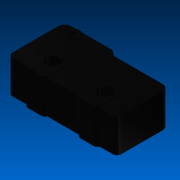
# Autodesk Inventor part: Omron SS-01GL2-E Microswitch Housing
Saved by Autodesk Inventor 2013 (Build 170138000, 138)
## iProperties
Created: 2012-05-23
Material: ABS Plastic
Document SubType Name: Modeling
Designer: sdarley
Density: 1 g/cm^3
Project: Microswitch - Omron SS-01GL2-E
Description: Omron SS-01GL2-E Microswitch Housing
Author: sdarley
Title: Omron SS-01GL2-E Microswitch Housing
Revision Number: 1
Autodesk Inventor part; units mm, degrees
ref_plane "YZ Plane" through (0, 0, 0) normal (1, 0, 0) x (0, 1, 0)
ref_plane "XZ Plane" through (0, 0, 0) normal (0, 1, 0) x (-1, 0, 0)
ref_plane "XY Plane" through (0, 0, 0) normal (0, 0, 1) x (1, 0, 0)
sketch "Sketch1" plane through (0, 0, 0) normal (0, 0, 1) x (1, 0, 0)
  line L0 (-9.75, 5.15) -> (-1, 5.15)
  line L1 (-1, 5.15) -> (0, 4.35)
  line L2 (0, 4.35) -> (10.1, 4.35)
  line L3 (10.1, 4.35) -> (10.1, -5.15)
  line L4 (10.1, -5.15) -> (6.75, -5.15)
  line L5 (6.75, -5.15) -> (6.3375, -5.45)
  line L6 (6.3375, -5.45) -> (3.5375, -5.45)
  line L7 (3.5375, -5.45) -> (3.125, -5.15)
  line L8 (3.125, -5.15) -> (-2.775, -5.15)
  line L9 (-2.775, -5.15) -> (-3.1875, -5.45)
  line L10 (-3.1875, -5.45) -> (-5.9875, -5.45)
  line L11 (-5.9875, -5.45) -> (-6.4, -5.15)
  line L12 (-6.4, -5.15) -> (-9.75, -5.15)
  line L13 (-9.75, -5.15) -> (-9.75, 5.15)
  point P0 (0, 0)
  point P1 (-9.75, 0)
  dimension "d0" = 19.85
  dimension "d2" = 10.6
  dimension "d3" = 9.5
  dimension "d4" = 0.3
  dimension "d5" = 5.9
  dimension "d6" = 3.35
  dimension "d7" = 3.35
  dimension "d8" = 10.1
  dimension "d9" = 8.75
  dimension "d10" = 2.8
  constraints: 28 end point, 9 parallel, 4 horizontal alignment, 2 equal length, 1 horizontal, 1 midpoint, 1 perpendicular, 1 vertical alignment
  measures "d0" distance between parallel lines of L3 L13
  measures "d2" distance between parallel lines of L6 L0
  measures "d3" distance between parallel lines of L4 L2
  measures "d4" distance between parallel lines of L6 L4
  measures "d5" distance of L7.end L8.end
  measures "d6" distance from line of L3 L4.end
  measures "d7" distance from line of L11.end L13
  measures "d8" distance of L1.end L2.end
  measures "d9" distance of L0.start L0.end
  measures "d10" distance of L9.end L10.end
extrude "Extrusion1" add sketch "Sketch1" along normal mid plane 6.1
sketch "Sketch2" plane through (0, 0, 3.05) normal (0, 0, 1) x (1, 0, 0)
  line L0 (-1, 5.15) -> (-9.75, 5.15) projected
  line L1 (-9.75, 5.15) -> (-9.75, -5.15) projected
  line L2 (-9.75, -5.15) -> (-6.4, -5.15) projected
  line L3 (-6.4, -5.15) -> (-5.9875, -5.45) projected
  line L4 (-5.9875, -5.45) -> (-3.1875, -5.45) projected
  line L5 (-3.1875, -5.45) -> (-2.775, -5.15) projected
  line L6 (3.125, -5.15) -> (3.5375, -5.45) projected
  line L7 (3.5375, -5.45) -> (6.3375, -5.45) projected
  line L8 (6.3375, -5.45) -> (6.75, -5.15) projected
  line L9 (10.1, 4.35) -> (0, 4.35) projected
  line L10 (-6.4, -5.15) -> (-6.4, -2.2125)
  line L11 (-2.775, -2.2125) -> (-2.775, -5.15)
  line L12 (3.125, -5.15) -> (3.125, -2.2125)
  line L13 (6.75, -2.2125) -> (6.75, -5.15)
  arc A0 (-2.775, -2.2125) -> (-6.4, -2.2125) centre (-4.5875, -2.2125) ccw
  arc A1 (6.75, -2.2125) -> (3.125, -2.2125) centre (4.9375, -2.2125) ccw
  circle A2 centre (-6.95, 4.05) radius 1.1
  point P0 (0, 0)
  dimension "d14" = 4.75
  dimension "d15" = 2.2
  dimension "d16" = 1.7
  constraints: 8 end point, 5 tangent, 4 point on circle, 3 centre point, 3 parallel, 1 horizontal alignment, 1 perpendicular
  measures "d15" diameter of A2
  measures "d16" distance edge to line of A2 L1
extrude "Extrusion2" add sketch "Sketch2" along normal blind 0.15
mirror "Mirror1" about plane through (0, 0, 0) normal (0, 0, 1) of "Extrusion2"
sketch "Sketch3" plane through (0, 0, 3.2) normal (0, 0, 1) x (1, 0, 0)
  arc A0 (-2.775, -2.2125) -> (-6.4, -2.2125) centre (-4.5875, -2.2125) ccw projected
  line L0 (3.125, -5.15) -> (3.5375, -5.45) projected
  line L1 (3.5375, -5.45) -> (6.3375, -5.45) projected
  line L2 (6.3375, -5.45) -> (6.75, -5.15) projected
  line L3 (6.75, -5.15) -> (6.75, -2.2125) projected
  arc A1 (6.75, -2.2125) -> (3.125, -2.2125) centre (4.9375, -2.2125) ccw projected
  line L4 (3.125, -2.2125) -> (3.125, -5.15) projected
  circle A2 centre (-4.5875, -2.2125) radius 1.175
  circle A3 centre (4.9375, -2.2125) radius 1.175
  circle A4 centre (-6.95, 4.05) radius 1.1 projected
  line L5 (-7.35, 4.35) -> (-6.8, 4.35)
  line L6 (-6.8, 4.35) -> (-6.8, 3.35)
  line L7 (-6.8, 3.35) -> (-7.35, 3.35)
  line L8 (-7.35, 3.35) -> (-7.35, 4.35)
  line L9 (-1, 5.15) -> (-6.95, 5.15) projected
  line L10 (10.1, -5.15) -> (10.1, 4.35) projected
  point P0 (0, 0)
  dimension "d19" = 2.35
  dimension "d21" = 2.35
  dimension "d24" = 0.55
  dimension "d25" = 1
  dimension "d35" = 0.8
  dimension "d36" = 16.9
  constraints: 8 end point, 2 centre point, 2 coincident, 2 parallel, 1 horizontal, 1 perpendicular, 1 vertical alignment
  measures "d19" diameter of A2
  measures "d21" diameter of A3
  measures "d24" distance of L6.end L7.end
  measures "d25" distance of L5.end L6.end
  measures "d35" distance between parallel lines of L9 L5
  measures "d36" distance between parallel lines of L10 L6
extrude "Extrusion3" cut sketch "Sketch3" against normal through all contours A2 | A3 | L5 L6 L7 L8
sketch "Sketch4" plane through (-9.75, 5.15, 3.05) normal (0, 1, 0) x (1, 0, 0)
  line L0 (0, 6.1) -> (0, 0) projected
  line L1 (2.5, 5.2) -> (2.8, 5.2)
  line L2 (2.8, 5.2) -> (2.8, 0.9)
  line L3 (2.8, 0.9) -> (2.5, 0.9)
  line L4 (2.5, 0.9) -> (2.5, 5.2)
  line L5 (5.85, 4.65) -> (7.85, 4.65)
  line L6 (7.85, 4.65) -> (7.85, 1.45)
  line L7 (7.85, 1.45) -> (5.85, 1.45)
  line L8 (5.85, 1.45) -> (5.85, 4.65)
  point P0 (9.75, 3.05)
  point P1 (0, 3.05)
  point P2 (2.5, 3.05)
  point P3 (2.8, 3.05)
  point P4 (5.85, 3.05)
  dimension "d26" = 4.3
  dimension "d28" = 0.3
  dimension "d29" = 2.5
  dimension "d30" = 3.05
  dimension "d31" = 2
  dimension "d32" = 3.2
  constraints: 16 end point, 4 midpoint, 4 parallel, 2 horizontal, 2 horizontal alignment, 2 perpendicular
  measures "d26" distance of L3.end L1.start
  measures "d28" distance of L1.start L1.end
  measures "d29" distance between parallel lines of L0 L4
  measures "d30" distance between parallel lines of L8 L2
  measures "d31" distance between parallel lines of L8 L6
  measures "d32" distance of L5.end L6.end
extrude "Extrusion4" cut sketch "Sketch4" against normal up to surface (1.8 mm away)
fillet "Fillet1" radius 1.2 2 edges at (-9.75, 5.15, 0) (10.1, 4.35, 0)
fillet "Fillet2" radius 0.75 2 edges at (-9.75, -5.15, 0) (10.1, -5.15, 0)
fillet "Fillet3" radius 0.3 10 edges at (0, 4.35, 0) (-1, 5.15, 0) (-2.775, -5.15, 0) (-3.1875, -5.45, 0) (-5.9875, -5.45, 0) (-6.4, -5.15, 0) (3.125, -5.15, 0) (3.5375, -5.45, 0) (6.3375, -5.45, 0) (6.75, -5.15, 0)
sketch "Sketch5" plane through (0, 0, 3.05) normal (0, 0, 1) x (1, 0, 0)
  line L0 (-9, -5.15) -> (-6.4976, -5.15) projected
  line L1 (-2.6774, -5.15) -> (3.0274, -5.15) projected
  line L2 (-8.5414, -3.4705) -> (-7.3088, -3.4705) construction
  line L3 (-7.3088, -3.4705) -> (-7.3088, -5.15) construction
  line L4 (-7.3088, -5.15) -> (-8.5414, -5.15) construction
  line L5 (-8.5414, -5.15) -> (-8.5414, -3.4705) construction
  line L6 (0.0618, -3.4705) -> (2.7283, -3.4705) construction
  line L7 (2.7283, -3.4705) -> (2.7283, -5.15) construction
  line L8 (2.7283, -5.15) -> (0.0618, -5.15) construction
  line L9 (0.0618, -5.15) -> (0.0618, -3.4705) construction
  line L10 (7.3318, -3.4705) -> (9.7732, -3.4705) construction
  line L11 (9.7732, -3.4705) -> (9.7732, -5.15) construction
  line L12 (9.7732, -5.15) -> (7.3318, -5.15) construction
  line L13 (7.3318, -5.15) -> (7.3318, -3.4705) construction
  spline S0 degree 2 poles (-7.8527, -4.9205) (-7.9889, -4.9205) (-8.2192, -4.8286) (-8.3032, -4.7367) knots 0 0 0 1 2 2 2
  spline S1 degree 2 poles (-8.3032, -4.7367) (-8.3871, -4.6459) (-8.479, -4.3736) (-8.479, -4.1966) knots 0 0 0 1 2 2 2
  spline S2 degree 2 poles (-8.479, -4.1966) (-8.479, -4.0208) (-8.3894, -3.7598) (-8.3043, -3.6634) knots 0 0 0 1 2 2 2
  spline S3 degree 2 poles (-8.3043, -3.6634) (-8.2203, -3.5692) (-7.9912, -3.4705) (-7.8493, -3.4705) knots 0 0 0 1 2 2 2
  spline S4 degree 2 poles (-7.8493, -3.4705) (-7.779, -3.4705) (-7.6553, -3.491) (-7.6032, -3.5068) knots 0 0 0 1 2 2 2
  spline S5 degree 2 poles (-7.6032, -3.5068) (-7.5578, -3.5216) (-7.4636, -3.5636) (-7.4171, -3.5885) knots 0 0 0 1 2 2 2
  line L14 (-7.4171, -3.5885) -> (-7.4171, -3.8132)
  line L15 (-7.4171, -3.8132) -> (-7.4318, -3.8132)
  spline S6 degree 2 poles (-7.4318, -3.8132) (-7.4568, -3.7905) (-7.5339, -3.7269) (-7.5895, -3.6963) knots 0 0 0 1 2 2 2
  spline S7 degree 2 poles (-7.5895, -3.6963) (-7.6429, -3.6668) (-7.7688, -3.6294) (-7.8505, -3.6294) knots 0 0 0 1 2 2 2
  spline S8 degree 2 poles (-7.8505, -3.6294) (-7.9401, -3.6294) (-8.1001, -3.7031) (-8.1602, -3.7735) knots 0 0 0 1 2 2 2
  spline S9 degree 2 poles (-8.1602, -3.7735) (-8.2192, -3.8449) (-8.285, -4.0616) (-8.285, -4.1966) knots 0 0 0 1 2 2 2
  spline S10 degree 2 poles (-8.285, -4.1966) (-8.285, -4.3407) (-8.2158, -4.5483) (-8.1557, -4.6198) knots 0 0 0 1 2 2 2
  spline S11 degree 2 poles (-8.1557, -4.6198) (-8.0967, -4.689) (-7.939, -4.7594) (-7.8505, -4.7594) knots 0 0 0 1 2 2 2
  spline S12 degree 2 poles (-7.8505, -4.7594) (-7.7699, -4.7594) (-7.6326, -4.7196) (-7.5793, -4.6901) knots 0 0 0 1 2 2 2
  spline S13 degree 2 poles (-7.5793, -4.6901) (-7.5283, -4.6606) (-7.4523, -4.5994) (-7.4307, -4.5778) knots 0 0 0 1 2 2 2
  line L16 (-7.4307, -4.5778) -> (-7.4171, -4.5778)
  line L17 (-7.4171, -4.5778) -> (-7.4171, -4.8002)
  spline S14 degree 2 poles (-7.4171, -4.8002) (-7.4636, -4.8217) (-7.5453, -4.8615) (-7.6032, -4.8796) knots 0 0 0 1 2 2 2
  spline S15 degree 2 poles (-7.6032, -4.8796) (-7.6644, -4.9) (-7.7688, -4.9205) (-7.8527, -4.9205) knots 0 0 0 1 2 2 2
  line L18 (1.2054, -4.9) -> (0.9966, -4.9)
  line L19 (0.9966, -4.9) -> (0.3772, -3.6929)
  line L20 (0.3772, -3.6929) -> (0.3772, -4.9)
  line L21 (0.3772, -4.9) -> (0.2036, -4.9)
  line L22 (0.2036, -4.9) -> (0.2036, -3.5)
  line L23 (0.2036, -3.5) -> (0.468, -3.5)
  line L24 (0.468, -3.5) -> (1.0318, -4.6085)
  line L25 (1.0318, -4.6085) -> (1.0318, -3.5)
  line L26 (1.0318, -3.5) -> (1.2054, -3.5)
  line L27 (1.2054, -3.5) -> (1.2054, -4.9)
  spline S16 degree 2 poles (2.4795, -3.66) (2.5589, -3.753) (2.6474, -4.0253) (2.6474, -4.2) knots 0 0 0 1 2 2 2
  spline S17 degree 2 poles (2.6474, -4.2) (2.6474, -4.3702) (2.5612, -4.6459) (2.4795, -4.7389) knots 0 0 0 1 2 2 2
  spline S18 degree 2 poles (2.4795, -4.7389) (2.3932, -4.8365) (2.1652, -4.9295) (2.0279, -4.9295) knots 0 0 0 1 2 2 2
  spline S19 degree 2 poles (2.0279, -4.9295) (1.8861, -4.9295) (1.6592, -4.8331) (1.5764, -4.7389) knots 0 0 0 1 2 2 2
  spline S20 degree 2 poles (1.5764, -4.7389) (1.4958, -4.6459) (1.4096, -4.3725) (1.4096, -4.2) knots 0 0 0 1 2 2 2
  spline S21 degree 2 poles (1.4096, -4.2) (1.4096, -4.0242) (1.497, -3.7564) (1.5775, -3.66) knots 0 0 0 1 2 2 2
  spline S22 degree 2 poles (1.5775, -3.66) (1.6592, -3.567) (1.8872, -3.4705) (2.0279, -3.4705) knots 0 0 0 1 2 2 2
  spline S23 degree 2 poles (2.0279, -3.4705) (2.1709, -3.4705) (2.4, -3.5704) (2.4795, -3.66) knots 0 0 0 1 2 2 2
  spline S24 degree 2 poles (2.4534, -4.2) (2.4534, -4.0616) (2.3932, -3.8472) (2.3388, -3.7769) knots 0 0 0 1 2 2 2
  spline S25 degree 2 poles (2.3388, -3.7769) (2.2832, -3.7042) (2.1266, -3.6316) (2.0291, -3.6316) knots 0 0 0 1 2 2 2
  spline S26 degree 2 poles (2.0291, -3.6316) (1.9281, -3.6316) (1.7761, -3.702) (1.7182, -3.7769) knots 0 0 0 1 2 2 2
  spline S27 degree 2 poles (1.7182, -3.7769) (1.6626, -3.8483) (1.6036, -4.0639) (1.6036, -4.2) knots 0 0 0 1 2 2 2
  spline S28 degree 2 poles (1.6036, -4.2) (1.6036, -4.4757) (1.8351, -4.7684) (2.0291, -4.7684) knots 0 0 0 1 2 2 2
  spline S29 degree 2 poles (2.0291, -4.7684) (2.2231, -4.7684) (2.4534, -4.4757) (2.4534, -4.2) knots 0 0 0 1 2 2 2
  line L28 (8.4754, -4.8955) -> (8.2666, -4.8955)
  line L29 (8.2666, -4.8955) -> (7.6472, -3.6884)
  line L30 (7.6472, -3.6884) -> (7.6472, -4.8955)
  line L31 (7.6472, -4.8955) -> (7.4736, -4.8955)
  line L32 (7.4736, -4.8955) -> (7.4736, -3.4955)
  line L33 (7.4736, -3.4955) -> (7.7379, -3.4955)
  line L34 (7.7379, -3.4955) -> (8.3018, -4.6039)
  line L35 (8.3018, -4.6039) -> (8.3018, -3.4955)
  line L36 (8.3018, -3.4955) -> (8.4754, -3.4955)
  line L37 (8.4754, -3.4955) -> (8.4754, -4.8955)
  spline S30 degree 2 poles (9.3058, -4.9205) (9.1697, -4.9205) (8.9394, -4.8286) (8.8554, -4.7367) knots 0 0 0 1 2 2 2
  spline S31 degree 2 poles (8.8554, -4.7367) (8.7715, -4.6459) (8.6796, -4.3736) (8.6796, -4.1966) knots 0 0 0 1 2 2 2
  spline S32 degree 2 poles (8.6796, -4.1966) (8.6796, -4.0208) (8.7692, -3.7598) (8.8543, -3.6634) knots 0 0 0 1 2 2 2
  spline S33 degree 2 poles (8.8543, -3.6634) (8.9382, -3.5692) (9.1674, -3.4705) (9.3092, -3.4705) knots 0 0 0 1 2 2 2
  spline S34 degree 2 poles (9.3092, -3.4705) (9.3796, -3.4705) (9.5032, -3.491) (9.5554, -3.5068) knots 0 0 0 1 2 2 2
  spline S35 degree 2 poles (9.5554, -3.5068) (9.6008, -3.5216) (9.695, -3.5636) (9.7415, -3.5885) knots 0 0 0 1 2 2 2
  line L38 (9.7415, -3.5885) -> (9.7415, -3.8132)
  line L39 (9.7415, -3.8132) -> (9.7267, -3.8132)
  spline S36 degree 2 poles (9.7267, -3.8132) (9.7018, -3.7905) (9.6246, -3.7269) (9.569, -3.6963) knots 0 0 0 1 2 2 2
  spline S37 degree 2 poles (9.569, -3.6963) (9.5157, -3.6668) (9.3898, -3.6294) (9.3081, -3.6294) knots 0 0 0 1 2 2 2
  spline S38 degree 2 poles (9.3081, -3.6294) (9.2185, -3.6294) (9.0585, -3.7031) (8.9984, -3.7735) knots 0 0 0 1 2 2 2
  spline S39 degree 2 poles (8.9984, -3.7735) (8.9394, -3.8449) (8.8736, -4.0616) (8.8736, -4.1966) knots 0 0 0 1 2 2 2
  spline S40 degree 2 poles (8.8736, -4.1966) (8.8736, -4.3407) (8.9428, -4.5483) (9.0029, -4.6198) knots 0 0 0 1 2 2 2
  spline S41 degree 2 poles (9.0029, -4.6198) (9.0619, -4.689) (9.2196, -4.7594) (9.3081, -4.7594) knots 0 0 0 1 2 2 2
  spline S42 degree 2 poles (9.3081, -4.7594) (9.3886, -4.7594) (9.5259, -4.7196) (9.5792, -4.6901) knots 0 0 0 1 2 2 2
  spline S43 degree 2 poles (9.5792, -4.6901) (9.6303, -4.6606) (9.7063, -4.5994) (9.7279, -4.5778) knots 0 0 0 1 2 2 2
  line L40 (9.7279, -4.5778) -> (9.7415, -4.5778)
  line L41 (9.7415, -4.5778) -> (9.7415, -4.8002)
  spline S44 degree 2 poles (9.7415, -4.8002) (9.695, -4.8217) (9.6133, -4.8615) (9.5554, -4.8796) knots 0 0 0 1 2 2 2
  spline S45 degree 2 poles (9.5554, -4.8796) (9.4942, -4.9) (9.3898, -4.9205) (9.3058, -4.9205) knots 0 0 0 1 2 2 2
  point P0 (0, 0)
  constraints: 3 horizontal alignment, 2 point on line, 6 other
extrude "Extrusion5" add sketch "Sketch5" along normal blind 0.05
sketch "Sketch6" plane through (0, 0, -3.05) normal (0, 0, -1) x (-1, 0, 0)
  arc A0 (-0.1052, 4.35) -> (0.0822, 4.4157) centre (-0.1052, 4.65) ccw projected
  line L0 (-0.0059, 4.3669) -> (7.1408, 4.3669) construction
  line L1 (7.1408, 4.3669) -> (7.1408, 2.1169) construction
  line L2 (7.1408, 2.1169) -> (-0.0059, 2.1169) construction
  line L3 (-0.0059, 2.1169) -> (-0.0059, 4.3669) construction
  line L4 (-10.1, 3.15) -> (-10.1, -4.4) projected
  line L5 (-9.35, -5.15) -> (-6.8476, -5.15) projected
  line L6 (-3.0274, -5.15) -> (2.6774, -5.15) projected
  line L7 (9.75, -4.4) -> (9.75, 3.95) projected
  line L8 (-9.1339, -3.4715) -> (-8.1314, -3.4715) construction
  line L9 (-8.1314, -3.4715) -> (-8.1314, -4.8125) construction
  line L10 (-8.1314, -4.8125) -> (-9.1339, -4.8125) construction
  line L11 (-9.1339, -4.8125) -> (-9.1339, -3.4715) construction
  line L12 (-2.1546, -3.4715) -> (-1.2541, -3.4715) construction
  line L13 (-1.2541, -3.4715) -> (-1.2541, -4.8125) construction
  line L14 (-1.2541, -4.8125) -> (-2.1546, -4.8125) construction
  line L15 (-2.1546, -4.8125) -> (-2.1546, -3.4715) construction
  line L16 (7.4519, -3.4715) -> (8.3839, -3.4715) construction
  line L17 (8.3839, -3.4715) -> (8.3839, -4.8125) construction
  line L18 (8.3839, -4.8125) -> (7.4519, -4.8125) construction
  line L19 (7.4519, -4.8125) -> (7.4519, -3.4715) construction
  line L20 (-8.9, -3.15) -> (-8.5, -3.15)
  line L21 (-8.5, -3.15) -> (-8.5, 0.2)
  line L22 (-8.5, 0.2) -> (-2, 0.2)
  line L23 (-8.9, -3.15) -> (-8.9, 0.6)
  line L24 (-8.9, 0.6) -> (-1.6, 0.6)
  line L25 (-0.0393, -1.1) -> (2.55, -1.1)
  line L26 (2.55, -1.1) -> (2.55, -1.5)
  line L27 (2.55, -1.5) -> (-0.1, -1.5)
  line L28 (5.8899, -5.45) -> (3.2851, -5.45) projected
  line L29 (-1.6, 0.6) -> (-1.6, -0.3)
  line L30 (-1.6, -0.3) -> (-1.5113, -0.3)
  line L31 (-1.5113, -0.3) -> (-1.8, -0.8)
  line L32 (-2, 0.2) -> (-2, -0.3)
  line L33 (-2, -0.3) -> (-2.0887, -0.3)
  line L34 (-2.0887, -0.3) -> (-1.8, -0.8)
  line L35 (-0.0393, -1.1) -> (-2.1313, -0.45)
  line L36 (-2.1313, -0.45) -> (-2.25, -0.832)
  line L37 (-2.25, -0.832) -> (-0.1, -1.5)
  line L38 (-3.6351, -5.45) -> (-6.2399, -5.45) projected
  line L39 (6.85, -1.1) -> (6.85, -1.5)
  line L40 (6.85, -1.5) -> (7.7, -1.5)
  line L41 (7.7, -1.5) -> (7.7, -3.15)
  line L42 (7.7, -3.15) -> (8.1, -3.15)
  line L43 (8.1, -3.15) -> (8.1, -1.1)
  line L44 (8.1, -1.1) -> (6.85, -1.1)
  line L45 (-1.6, -3.15) -> (-2, -3.15)
  line L46 (-2, -3.15) -> (-2, -2.333)
  line L47 (-2, -2.333) -> (-2.05, -2.333)
  line L48 (-2.05, -2.333) -> (-1.8, -1.9)
  line L49 (-1.8, -1.9) -> (-1.55, -2.333)
  line L50 (-1.55, -2.333) -> (-1.6, -2.333)
  line L51 (-1.6, -2.333) -> (-1.6, -3.15)
  line L52 (0.9178, 5.0843) -> (0.0822, 4.4157) projected
  circle A1 centre (-7.7959, 3.0628) radius 0.4188
  circle A2 centre (-7.7959, 3.0628) radius 0.7
  circle A3 centre (-3.3347, 3.0628) radius 0.4188
  circle A4 centre (-3.3347, 3.0628) radius 0.7
  line L53 (-6.98, 3.7628) -> (-6.98, 2.3628)
  line L54 (-6.98, 2.3628) -> (-6.7014, 2.3628)
  line L55 (-6.7014, 3.4816) -> (-6.7014, 2.3628)
  line L56 (-6.7014, 3.4816) -> (-6.3607, 3.4816)
  line L57 (-6.3607, 3.4816) -> (-6.3607, 2.3628)
  line L58 (-6.0774, 2.3628) -> (-6.0774, 3.4816)
  line L59 (-6.0774, 3.4816) -> (-5.8769, 3.4816)
  line L60 (-6.98, 3.7628) -> (-5.8746, 3.7628)
  line L61 (-6.3607, 2.3628) -> (-6.0774, 2.3628)
  line L62 (-5.7287, 2.3628) -> (-5.7287, 3.3334)
  line L63 (-5.7287, 2.3628) -> (-5.4364, 2.3628)
  line L64 (-5.4364, 2.3628) -> (-5.4364, 3.2892)
  line L65 (-5.272, 3.7628) -> (-5.272, 2.3628)
  line L66 (-5.272, 2.3628) -> (-4.9837, 2.3628)
  line L67 (-4.9837, 2.3628) -> (-4.9837, 3.5038)
  line L68 (-5.272, 3.7628) -> (-4.5256, 3.7628)
  line L69 (-4.4487, 2.8778) -> (-4.0366, 2.3628)
  line L70 (-4.3901, 2.3628) -> (-4.0366, 2.3628)
  line L71 (-4.3901, 2.3628) -> (-4.8491, 3.0137)
  line L72 (-4.9837, 3.5038) -> (-4.6228, 3.5038)
  arc A5 (-5.4364, 3.2892) -> (-5.8746, 3.7628) centre (-5.9114, 3.2892) ccw
  arc A6 (-5.7287, 3.3334) -> (-5.8769, 3.4816) centre (-5.8769, 3.3334) ccw
  arc A7 (-4.5825, 3.0628) -> (-4.6228, 3.5038) centre (-4.6228, 3.2815) ccw
  arc A8 (-4.4487, 2.8778) -> (-4.5256, 3.7628) centre (-4.5825, 3.312) ccw
  line L73 (-4.8491, 3.0137) -> (-4.5825, 3.0628)
  line L74 (-2.5151, 2.3628) -> (-2.5151, 2.443)
  line L75 (-2.5151, 2.443) -> (-2.5151, 3.7628)
  line L76 (-2.5151, 3.7628) -> (-1.836, 3.7628)
  line L77 (-2.5151, 2.3628) -> (-2.2307, 2.3628)
  line L78 (-2.2307, 3.5038) -> (-2.2307, 2.3628)
  line L79 (-2.2307, 3.5038) -> (-1.869, 3.5038)
  line L80 (-1.675, 2.3628) -> (-1.675, 3.3098)
  line L81 (-1.675, 2.3628) -> (-1.4257, 2.3628)
  line L82 (-1.4257, 2.3628) -> (-1.4257, 3.3525)
  arc A9 (-1.675, 3.3098) -> (-1.869, 3.5038) centre (-1.869, 3.3098) ccw
  arc A10 (-1.4257, 3.3525) -> (-1.836, 3.7628) centre (-1.836, 3.3525) ccw
  line L83 (0.0726, 3.3669) -> (0.0726, 4.3669)
  line L84 (0.0726, 4.3669) -> (0.2212, 4.3669)
  line L85 (0.2212, 4.3669) -> (0.3988, 3.6588)
  spline S0 degree 2 poles (0.3988, 3.6588) (0.4232, 3.5597) (0.4346, 3.511) knots 0 0 0 1 1 1
  spline S1 degree 2 poles (0.4346, 3.511) (0.4468, 3.5651) (0.4743, 3.671) knots 0 0 0 1 1 1
  line L86 (0.4743, 3.671) -> (0.6541, 4.3669)
  line L87 (0.6541, 4.3669) -> (0.7868, 4.3669)
  line L88 (0.7868, 4.3669) -> (0.7868, 3.3669)
  line L89 (0.7868, 3.3669) -> (0.6915, 3.3669)
  line L90 (0.6915, 3.3669) -> (0.6915, 4.2038)
  line L91 (0.6915, 4.2038) -> (0.4735, 3.3669)
  line L92 (0.4735, 3.3669) -> (0.3843, 3.3669)
  line L93 (0.3843, 3.3669) -> (0.1678, 4.2183)
  line L94 (0.1678, 4.2183) -> (0.1678, 3.3669)
  line L95 (0.1678, 3.3669) -> (0.0726, 3.3669)
  line L96 (0.8645, 3.3669) -> (1.1518, 4.3669)
  line L97 (1.1518, 4.3669) -> (1.2593, 4.3669)
  line L98 (1.2593, 4.3669) -> (1.5657, 3.3669)
  line L99 (1.5657, 3.3669) -> (1.4529, 3.3669)
  line L100 (1.4529, 3.3669) -> (1.366, 3.6695)
  line L101 (1.366, 3.6695) -> (1.052, 3.6695)
  line L102 (1.052, 3.6695) -> (0.9697, 3.3669)
  line L103 (0.9697, 3.3669) -> (0.8645, 3.3669)
  line L104 (1.0802, 3.777) -> (1.3355, 3.777)
  line L105 (1.3355, 3.777) -> (1.257, 4.0544)
  spline S2 degree 2 poles (1.257, 4.0544) (1.2212, 4.1809) (1.2037, 4.2617) knots 0 0 0 1 1 1
  spline S3 degree 2 poles (1.2037, 4.2617) (1.1884, 4.1657) (1.1633, 4.0712) knots 0 0 0 1 1 1
  line L106 (1.1633, 4.0712) -> (1.0802, 3.777)
  line L107 (1.645, 3.3669) -> (1.645, 4.3669)
  line L108 (1.645, 4.3669) -> (1.9034, 4.3669)
  spline S4 degree 2 poles (1.9034, 4.3669) (1.9903, 4.3669) (2.0368, 4.3524) knots 0 0 0 1 1 1
  spline S5 degree 2 poles (2.0368, 4.3524) (2.1008, 4.3326) (2.1465, 4.2808) knots 0 0 0 1 1 1
  spline S6 degree 2 poles (2.1465, 4.2808) (2.206, 4.2145) (2.2646, 4.0064) (2.2646, 3.8722) knots 0 0 0 1 2 2 2
  spline S7 degree 2 poles (2.2646, 3.8722) (2.2646, 3.7587) (2.225, 3.5826) (2.1625, 3.4675) (2.0886, 3.4012) (1.9834, 3.3669) (1.9156, 3.3669) knots 0 0 0 1 2 3 4 5 5 5
  line L109 (1.9156, 3.3669) -> (1.645, 3.3669)
  line L110 (1.7441, 3.4851) -> (1.9041, 3.4851)
  spline S8 degree 2 poles (1.9041, 3.4851) (1.9781, 3.4851) (2.0627, 3.5216) (2.0878, 3.5552) knots 0 0 0 1 2 2 2
  spline S9 degree 2 poles (2.0878, 3.5552) (2.1229, 3.6024) (2.1625, 3.761) (2.1625, 3.8745) knots 0 0 0 1 2 2 2
  spline S10 degree 2 poles (2.1625, 3.8745) (2.1625, 4.0315) (2.0855, 4.2) (2.0299, 4.2282) knots 0 0 0 1 2 2 2
  spline S11 degree 2 poles (2.0299, 4.2282) (1.9903, 4.2488) (1.9018, 4.2488) knots 0 0 0 1 1 1
  line L111 (1.9018, 4.2488) -> (1.7441, 4.2488)
  line L112 (1.7441, 4.2488) -> (1.7441, 3.4851)
  line L113 (2.4026, 3.3669) -> (2.4026, 4.3669)
  line L114 (2.4026, 4.3669) -> (2.9438, 4.3669)
  line L115 (2.9438, 4.3669) -> (2.9438, 4.2488)
  line L116 (2.9438, 4.2488) -> (2.5017, 4.2488)
  line L117 (2.5017, 4.2488) -> (2.5017, 3.9431)
  line L118 (2.5017, 3.9431) -> (2.9156, 3.9431)
  line L119 (2.9156, 3.9431) -> (2.9156, 3.825)
  line L120 (2.9156, 3.825) -> (2.5017, 3.825)
  line L121 (2.5017, 3.825) -> (2.5017, 3.4851)
  line L122 (2.5017, 3.4851) -> (2.9613, 3.4851)
  line L123 (2.9613, 3.4851) -> (2.9613, 3.3669)
  line L124 (2.9613, 3.3669) -> (2.4026, 3.3669)
  line L125 (3.4057, 3.3669) -> (3.4057, 4.3669)
  line L126 (3.4057, 4.3669) -> (3.5047, 4.3669)
  line L127 (3.5047, 4.3669) -> (3.5047, 3.3669)
  line L128 (3.5047, 3.3669) -> (3.4057, 3.3669)
  line L129 (3.6785, 3.3669) -> (3.6785, 4.3669)
  line L130 (3.6785, 4.3669) -> (3.7807, 4.3669)
  line L131 (3.7807, 4.3669) -> (4.1732, 3.5819)
  line L132 (4.1732, 3.5819) -> (4.1732, 4.3669)
  line L133 (4.1732, 4.3669) -> (4.2685, 4.3669)
  line L134 (4.2685, 4.3669) -> (4.2685, 3.3669)
  line L135 (4.2685, 3.3669) -> (4.1663, 3.3669)
  line L136 (4.1663, 3.3669) -> (3.7738, 4.152)
  line L137 (3.7738, 4.152) -> (3.7738, 3.3669)
  line L138 (3.7738, 3.3669) -> (3.6785, 3.3669)
  line L139 (0.0916, 2.1669) -> (0.0916, 3.1669)
  line L140 (0.0916, 3.1669) -> (0.1907, 3.1669)
  line L141 (0.1907, 3.1669) -> (0.1907, 2.1669)
  line L142 (0.1907, 2.1669) -> (0.0916, 2.1669)
  line L143 (0.3645, 2.1669) -> (0.3645, 3.1669)
  line L144 (0.3645, 3.1669) -> (0.4666, 3.1669)
  line L145 (0.4666, 3.1669) -> (0.8592, 2.3819)
  line L146 (0.8592, 2.3819) -> (0.8592, 3.1669)
  line L147 (0.8592, 3.1669) -> (0.9544, 3.1669)
  line L148 (0.9544, 3.1669) -> (0.9544, 2.1669)
  line L149 (0.9544, 2.1669) -> (0.8523, 2.1669)
  line L150 (0.8523, 2.1669) -> (0.4598, 2.952)
  line L151 (0.4598, 2.952) -> (0.4598, 2.1669)
  line L152 (0.4598, 2.1669) -> (0.3645, 2.1669)
  line L153 (1.1206, 2.1669) -> (1.1206, 3.1669)
  line L154 (1.1206, 3.1669) -> (1.379, 3.1669)
  spline S12 degree 2 poles (1.379, 3.1669) (1.4659, 3.1669) (1.5124, 3.1524) knots 0 0 0 1 1 1
  spline S13 degree 2 poles (1.5124, 3.1524) (1.5764, 3.1326) (1.6221, 3.0808) knots 0 0 0 1 1 1
  spline S14 degree 2 poles (1.6221, 3.0808) (1.6816, 3.0145) (1.7403, 2.8064) (1.7403, 2.6722) knots 0 0 0 1 2 2 2
  spline S15 degree 2 poles (1.7403, 2.6722) (1.7403, 2.5587) (1.7006, 2.3826) (1.6381, 2.2675) (1.5642, 2.2012) (1.459, 2.1669) (1.3912, 2.1669) knots 0 0 0 1 2 3 4 5 5 5
  line L155 (1.3912, 2.1669) -> (1.1206, 2.1669)
  line L156 (1.2197, 2.2851) -> (1.3797, 2.2851)
  spline S16 degree 2 poles (1.3797, 2.2851) (1.4537, 2.2851) (1.5383, 2.3216) (1.5634, 2.3552) knots 0 0 0 1 2 2 2
  spline S17 degree 2 poles (1.5634, 2.3552) (1.5985, 2.4024) (1.6381, 2.561) (1.6381, 2.6745) knots 0 0 0 1 2 2 2
  spline S18 degree 2 poles (1.6381, 2.6745) (1.6381, 2.8315) (1.5611, 3) (1.5055, 3.0282) knots 0 0 0 1 2 2 2
  spline S19 degree 2 poles (1.5055, 3.0282) (1.4659, 3.0488) (1.3775, 3.0488) knots 0 0 0 1 1 1
  line L157 (1.3775, 3.0488) -> (1.2197, 3.0488)
  line L158 (1.2197, 3.0488) -> (1.2197, 2.2851)
  spline S20 degree 2 poles (1.8454, 2.654) (1.8454, 2.9032) (2.0459, 3.1844) (2.2044, 3.1844) knots 0 0 0 1 2 2 2
  spline S21 degree 2 poles (2.2044, 3.1844) (2.3081, 3.1844) (2.4743, 3.0518) (2.5619, 2.8155) (2.5619, 2.6654) knots 0 0 0 1 2 3 3 3
  spline S22 degree 2 poles (2.5619, 2.6654) (2.5619, 2.5137) (2.4697, 2.2736) (2.3012, 2.1501) (2.2037, 2.1501) knots 0 0 0 1 2 3 3 3
  spline S23 degree 2 poles (2.2037, 2.1501) (2.0977, 2.1501) (1.9316, 2.2866) (1.8454, 2.5221) (1.8454, 2.654) knots 0 0 0 1 2 3 3 3
  spline S24 degree 2 poles (1.9476, 2.6524) (1.9476, 2.4718) (2.0932, 2.2637) (2.2029, 2.2637) knots 0 0 0 1 2 2 2
  spline S25 degree 2 poles (2.2029, 2.2637) (2.315, 2.2637) (2.4598, 2.4733) (2.4598, 2.6669) knots 0 0 0 1 2 2 2
  spline S26 degree 2 poles (2.4598, 2.6669) (2.4598, 2.7889) (2.398, 2.971) (2.2791, 3.0709) (2.2044, 3.0709) knots 0 0 0 1 2 3 3 3
  spline S27 degree 2 poles (2.2044, 3.0709) (2.0993, 3.0709) (1.9476, 2.878) (1.9476, 2.6524) knots 0 0 0 1 2 2 2
  line L159 (2.6892, 2.1669) -> (2.6892, 3.1669)
  line L160 (2.6892, 3.1669) -> (2.7913, 3.1669)
  line L161 (2.7913, 3.1669) -> (3.1839, 2.3819)
  line L162 (3.1839, 2.3819) -> (3.1839, 3.1669)
  line L163 (3.1839, 3.1669) -> (3.2791, 3.1669)
  line L164 (3.2791, 3.1669) -> (3.2791, 2.1669)
  line L165 (3.2791, 2.1669) -> (3.177, 2.1669)
  line L166 (3.177, 2.1669) -> (2.7845, 2.952)
  line L167 (2.7845, 2.952) -> (2.7845, 2.1669)
  line L168 (2.7845, 2.1669) -> (2.6892, 2.1669)
  line L169 (3.4476, 2.1669) -> (3.4476, 3.1669)
  line L170 (3.4476, 3.1669) -> (3.9887, 3.1669)
  line L171 (3.9887, 3.1669) -> (3.9887, 3.0488)
  line L172 (3.9887, 3.0488) -> (3.5467, 3.0488)
  line L173 (3.5467, 3.0488) -> (3.5467, 2.7431)
  line L174 (3.5467, 2.7431) -> (3.9605, 2.7431)
  line L175 (3.9605, 2.7431) -> (3.9605, 2.625)
  line L176 (3.9605, 2.625) -> (3.5467, 2.625)
  line L177 (3.5467, 2.625) -> (3.5467, 2.2851)
  line L178 (3.5467, 2.2851) -> (4.0063, 2.2851)
  line L179 (4.0063, 2.2851) -> (4.0063, 2.1669)
  line L180 (4.0063, 2.1669) -> (3.4476, 2.1669)
  line L181 (4.1107, 2.4886) -> (4.2044, 2.4992)
  spline S28 degree 2 poles (4.2044, 2.4992) (4.2113, 2.4238) (4.2593, 2.3277) (4.3614, 2.2683) (4.4255, 2.2683) knots 0 0 0 1 2 3 3 3
  spline S29 degree 2 poles (4.4255, 2.2683) (4.4819, 2.2683) (4.5688, 2.3133) (4.6107, 2.3918) (4.6107, 2.4383) knots 0 0 0 1 2 3 3 3
  spline S30 degree 2 poles (4.6107, 2.4383) (4.6107, 2.4855) (4.5688, 2.5556) (4.5223, 2.5793) knots 0 0 0 1 2 2 2
  spline S31 degree 2 poles (4.5223, 2.5793) (4.4918, 2.5953) (4.286, 2.6616) (4.2448, 2.6913) knots 0 0 0 1 2 2 2
  spline S32 degree 2 poles (4.2448, 2.6913) (4.1915, 2.7286) (4.1389, 2.8399) (4.1389, 2.9085) knots 0 0 0 1 2 2 2
  spline S33 degree 2 poles (4.1389, 2.9085) (4.1389, 2.9847) (4.2029, 3.1158) (4.3264, 3.1844) (4.4018, 3.1844) knots 0 0 0 1 2 3 3 3
  spline S34 degree 2 poles (4.4018, 3.1844) (4.4849, 3.1844) (4.6122, 3.1128) (4.6808, 2.9733) (4.6831, 2.8857) knots 0 0 0 1 2 3 3 3
  line L182 (4.6831, 2.8857) -> (4.5878, 2.8758)
  spline S35 degree 2 poles (4.5878, 2.8758) (4.5802, 2.971) (4.4918, 3.0678) (4.4057, 3.0678) knots 0 0 0 1 2 2 2
  spline S36 degree 2 poles (4.4057, 3.0678) (4.3165, 3.0678) (4.2342, 2.9794) (4.2342, 2.9177) knots 0 0 0 1 2 2 2
  spline S37 degree 2 poles (4.2342, 2.9177) (4.2342, 2.8636) (4.2631, 2.8285) knots 0 0 0 1 1 1
  spline S38 degree 2 poles (4.2631, 2.8285) (4.2921, 2.7942) (4.5329, 2.721) (4.5779, 2.6936) knots 0 0 0 1 2 2 2
  spline S39 degree 2 poles (4.5779, 2.6936) (4.6435, 2.6532) (4.706, 2.5297) (4.706, 2.4497) knots 0 0 0 1 2 2 2
  spline S40 degree 2 poles (4.706, 2.4497) (4.706, 2.3697) (4.6374, 2.2286) (4.5093, 2.1501) (4.4293, 2.1501) knots 0 0 0 1 2 3 3 3
  spline S41 degree 2 poles (4.4293, 2.1501) (4.3279, 2.1501) (4.1907, 2.2294) (4.113, 2.3879) (4.1107, 2.4886) knots 0 0 0 1 2 3 3 3
  line L183 (4.8584, 2.1669) -> (4.8584, 3.1669)
  line L184 (4.8584, 3.1669) -> (4.9575, 3.1669)
  line L185 (4.9575, 3.1669) -> (4.9575, 2.1669)
  line L186 (4.9575, 2.1669) -> (4.8584, 2.1669)
  line L187 (5.0497, 2.1669) -> (5.3371, 3.1669)
  line L188 (5.3371, 3.1669) -> (5.4445, 3.1669)
  line L189 (5.4445, 3.1669) -> (5.7509, 2.1669)
  line L190 (5.7509, 2.1669) -> (5.6381, 2.1669)
  line L191 (5.6381, 2.1669) -> (5.5512, 2.4695)
  line L192 (5.5512, 2.4695) -> (5.2372, 2.4695)
  line L193 (5.2372, 2.4695) -> (5.1549, 2.1669)
  line L194 (5.1549, 2.1669) -> (5.0497, 2.1669)
  line L195 (5.2654, 2.577) -> (5.5207, 2.577)
  line L196 (5.5207, 2.577) -> (5.4422, 2.8544)
  spline S42 degree 2 poles (5.4422, 2.8544) (5.4064, 2.9809) (5.3889, 3.0617) knots 0 0 0 1 1 1
  spline S43 degree 2 poles (5.3889, 3.0617) (5.3736, 2.9657) (5.3485, 2.8712) knots 0 0 0 1 1 1
  line L197 (5.3485, 2.8712) -> (5.2654, 2.577)
  line L198 (-8.2906, -4.5343) -> (-8.2906, -4.6761)
  line L199 (-8.2906, -4.6761) -> (-9.0836, -4.6761)
  spline S44 degree 2 poles (-9.0836, -4.6761) (-9.0855, -4.6231) (-9.0663, -4.5737) knots 0 0 0 1 1 1
  spline S45 degree 2 poles (-9.0663, -4.5737) (-9.0361, -4.4923) (-8.9025, -4.3359) (-8.7763, -4.2325) knots 0 0 0 1 2 2 2
  spline S46 degree 2 poles (-8.7763, -4.2325) (-8.5815, -4.0715) (-8.4443, -3.885) (-8.4443, -3.8008) knots 0 0 0 1 2 2 2
  spline S47 degree 2 poles (-8.4443, -3.8008) (-8.4443, -3.713) (-8.5696, -3.5932) (-8.6702, -3.5932) knots 0 0 0 1 2 2 2
  spline S48 degree 2 poles (-8.6702, -3.5932) (-8.7763, -3.5932) (-8.9035, -3.7212) (-8.9044, -3.8337) knots 0 0 0 1 2 2 2
  line L200 (-8.9044, -3.8337) -> (-9.0562, -3.8182)
  spline S49 degree 2 poles (-9.0562, -3.8182) (-9.0406, -3.649) (-8.8376, -3.4715) (-8.6666, -3.4715) knots 0 0 0 1 2 2 2
  spline S50 degree 2 poles (-8.6666, -3.4715) (-8.4937, -3.4715) (-8.2925, -3.6627) (-8.2925, -3.8045) knots 0 0 0 1 2 2 2
  spline S51 degree 2 poles (-8.2925, -3.8045) (-8.2925, -3.8767) (-8.351, -4.0158) (-8.4882, -4.1694) (-8.6464, -4.3039) knots 0 0 0 1 2 3 3 3
  spline S52 degree 2 poles (-8.6464, -4.3039) (-8.7791, -4.4145) (-8.8541, -4.4941) (-8.8788, -4.5343) knots 0 0 0 1 2 2 2
  line L201 (-8.8788, -4.5343) -> (-8.2906, -4.5343)
  line L202 (-2.0842, -4.3578) -> (-1.9369, -4.3386)
  spline S53 degree 2 poles (-1.9369, -4.3386) (-1.9113, -4.4639) (-1.7896, -4.5746) (-1.7018, -4.5746) knots 0 0 0 1 2 2 2
  spline S54 degree 2 poles (-1.7018, -4.5746) (-1.5976, -4.5746) (-1.4549, -4.4301) (-1.4549, -4.324) knots 0 0 0 1 2 2 2
  spline S55 degree 2 poles (-1.4549, -4.324) (-1.4549, -4.2225) (-1.5875, -4.0908) (-1.69, -4.0908) knots 0 0 0 1 2 2 2
  spline S56 degree 2 poles (-1.69, -4.0908) (-1.7311, -4.0908) (-1.7933, -4.1072) knots 0 0 0 1 1 1
  line L203 (-1.7933, -4.1072) -> (-1.7778, -3.9783)
  spline S57 degree 2 poles (-1.7778, -3.9783) (-1.7622, -3.9801) (-1.754, -3.9801) knots 0 0 0 1 1 1
  spline S58 degree 2 poles (-1.754, -3.9801) (-1.6598, -3.9801) (-1.5089, -3.8813) (-1.5089, -3.7798) knots 0 0 0 1 2 2 2
  spline S59 degree 2 poles (-1.5089, -3.7798) (-1.5089, -3.6984) (-1.6186, -3.5923) (-1.7055, -3.5923) knots 0 0 0 1 2 2 2
  spline S60 degree 2 poles (-1.7055, -3.5923) (-1.7915, -3.5923) (-1.9058, -3.7002) (-1.9223, -3.809) knots 0 0 0 1 2 2 2
  line L204 (-1.9223, -3.809) -> (-2.0695, -3.7825)
  spline S61 degree 2 poles (-2.0695, -3.7825) (-2.0421, -3.6343) (-1.8509, -3.4715) (-1.7082, -3.4715) knots 0 0 0 1 2 2 2
  spline S62 degree 2 poles (-1.7082, -3.4715) (-1.6104, -3.4715) (-1.4448, -3.5557) (-1.357, -3.7011) (-1.357, -3.7825) knots 0 0 0 1 2 3 3 3
  spline S63 degree 2 poles (-1.357, -3.7825) (-1.357, -3.8603) (-1.4403, -3.9883) (-1.5226, -4.0258) knots 0 0 0 1 2 2 2
  spline S64 degree 2 poles (-1.5226, -4.0258) (-1.4156, -4.0505) (-1.2985, -4.2051) (-1.2985, -4.3212) knots 0 0 0 1 2 2 2
  spline S65 degree 2 poles (-1.2985, -4.3212) (-1.2985, -4.4776) (-1.5281, -4.6962) (-1.7028, -4.6962) knots 0 0 0 1 2 2 2
  spline S66 degree 2 poles (-1.7028, -4.6962) (-1.861, -4.6962) (-2.0695, -4.5078) (-2.0842, -4.3578) knots 0 0 0 1 2 2 2
  line L205 (8.0757, -4.6761) -> (7.9284, -4.6761)
  line L206 (7.9284, -4.6761) -> (7.9284, -3.7377)
  spline S67 degree 2 poles (7.9284, -3.7377) (7.8754, -3.788) (7.7025, -3.8895) (7.6339, -3.9151) knots 0 0 0 1 2 2 2
  line L207 (7.6339, -3.9151) -> (7.6339, -3.7725)
  spline S68 degree 2 poles (7.6339, -3.7725) (7.7574, -3.7148) (7.9422, -3.5493) (7.9806, -3.4715) knots 0 0 0 1 2 2 2
  line L208 (7.9806, -3.4715) -> (8.0757, -3.4715)
  line L209 (8.0757, -3.4715) -> (8.0757, -4.6761)
  point P0 (0, 0)
  point P1 (-0.0059, 4.3669)
  dimension "d0" = 19.85
  dimension "d2" = 10.6
  dimension "d3" = 9.5
  dimension "d4" = 0.3
  dimension "d5" = 5.9
  dimension "d6" = 3.35
  dimension "d7" = 3.35
  dimension "d8" = 10.1
  dimension "d9" = 8.75
  dimension "d10" = 2.8
  dimension "d42" = 2.25
  dimension "d47" = 0.4
  dimension "d48" = 0.4
  dimension "d50" = 2
  dimension "d52" = 1.6
  dimension "d54" = 0.4
  dimension "d58" = 2.65
  dimension "d59" = 7.2
  dimension "d61" = 7.3
  dimension "d62" = 60
  dimension "d64" = 0.4
  dimension "d65" = 0.5
  dimension "d66" = 0.4
  dimension "d67" = 4.8
  dimension "d68" = 0.9
  dimension "d69" = 4.05
  dimension "d70" = 4.7
  dimension "d71" = 6.05
  dimension "d72" = 0.4
  dimension "d73" = 0.4
  dimension "d74" = 1.25
  dimension "d75" = 2.05
  dimension "d76" = 0.4
  dimension "d77" = 1.25
  dimension "d78" = 0.5
  constraints: 120 end point, 23 perpendicular, 15 parallel, 13 point on circle, 10 centre point, 9 tangent, 8 horizontal alignment, 4 equal length, 3 coincident, 1 equal radius, 1 vertical alignment, 8 other
  measures "d42" distance between parallel lines of L2 L0
  measures "d47" distance of L20.start L20.end
  measures "d48" distance between parallel lines of L24 L22
  measures "d50" distance between parallel lines of L20 L5
  measures "d52" distance between parallel lines of L4 L21
  measures "d54" distance of L25.end L26.end
  measures "d58" distance of L26.end L27.end
  measures "d59" distance between parallel lines of L7 L26
  measures "d61" distance of L23.end L24.end
  measures "d62" angle of L30 L31
  measures "d64" distance between parallel lines of L29 L32
  measures "d65" distance from line of L31.end L33
  measures "d66" distance of L35.end L36.end
  measures "d67" distance from line of L36.end L26
  measures "d68" distance between parallel lines of L33 L24
  measures "d69" distance between parallel lines of L25 L6
  measures "d70" distance from line of L6 L35.end
  measures "d71" distance between parallel lines of L38 L24
  measures "d72" distance between parallel lines of L44 L40
  measures "d73" distance between parallel lines of L43 L41
  measures "d74" distance between parallel lines of L43 L39
  measures "d75" distance between parallel lines of L7 L41
  measures "d76" distance of L45.start L45.end
  measures "d77" distance from line of L48.end L45
  measures "d78" distance of L49.end L47.end
extrude "Extrusion6" add sketch "Sketch6" along normal blind 0.05
equation "\"d7\" = d6"
equation "\"d21\" = d19"
equation "\"d48\" = d47"
equation "\"d54\" = d47"
equation "\"d64\" = d47"
equation "\"d65\" = d78"
equation "\"d72\" = d47"
equation "\"d73\" = d47"
equation "\"d76\" = d47"
body "Solid1"
